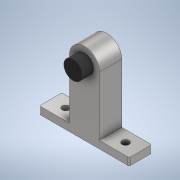
# Autodesk Inventor part: Stop sliding
Saved by Autodesk Inventor 2021 (Build 250183000, 183)
## iProperties
Created: 2021-06-07
Part Number: Stop sliding
Material: Generic
Document SubType Name: Modeling
Designer: Nelson
Density: 1 g/cm^3
Appearance: Default
Author: Nelson
Autodesk Inventor part; units mm, degrees
ref_plane "YZ Plane" through (0, 0, 0) normal (1, 0, 0) x (0, 1, 0)
ref_plane "XZ Plane" through (0, 0, 0) normal (0, 1, 0) x (-1, 0, 0)
ref_plane "XY Plane" through (0, 0, 0) normal (0, 0, 1) x (1, 0, 0)
sketch "Sketch3" plane through (0, 0, 0) normal (0, 0, 1) x (1, 0, 0)
  line L0 (0, 0) -> (60, 0)
  line L1 (60, 0) -> (60, 10)
  line L2 (60, 10) -> (20, 10)
  line L3 (20, 10) -> (20, 89)
  line L4 (0, 0) -> (0, 29.8306) construction
  line L5 (0, 0) -> (-60, 0)
  line L6 (-60, 0) -> (-60, 10)
  line L7 (-60, 10) -> (-20, 10)
  line L8 (-20, 10) -> (-20, 89)
  arc A0 (20, 89) -> (-20, 89) centre (0, 89) ccw
  dimension "d10" = 60
  dimension "d11" = 10
  dimension "d12" = 40
  dimension "d13" = 79
  dimension "d19" = 20
  constraints: 18 end point, 4 symmetric about line, 2 horizontal, 2 point on circle, 2 vertical, 1 centre point, 1 perpendicular
  measures "d10" distance of L0.start L0.end
  measures "d11" distance of L0.end L1.end
  measures "d12" distance of L1.end L2.end
  measures "d13" distance of L2.end L3.end
  measures "d19" radius of A0
extrude "Extrusion1" add sketch "Sketch3" against normal blind 30
sketch "Sketch4" plane through (0, 0, 0) normal (0, 0, 1) x (1, 0, 0)
  arc A0 (20, 89) -> (-20, 89) centre (0, 89) ccw projected
  circle A1 centre (0, 89) radius 12.5
  point P0 (0, 0)
  dimension "d20" = 25
  constraints: 1 centre point, 1 coincident
  measures "d20" diameter of A1
extrude "Extrusion2" add sketch "Sketch4" along normal blind 15
fillet "Fillet1" radius 2 4 edges at (60, 5, 0) (60, 5, -30) (-60, 5, 0) (-60, 5, -30)
sketch "Sketch5" plane through (-20, 10, 0) normal (0, 1, 0) x (1, 0, 0)
  line L0 (-38, 30) -> (0, 30) projected
  line L1 (40, 30) -> (78, 30) projected
  line L2 (-40, 2) -> (-40, 28) projected
  line L3 (80, 2) -> (80, 28) projected
  point P0 (20, 0)
  point P1 (-20, 15)
  point P2 (60, 15)
  dimension "d24" = 15
  dimension "d25" = 15
  dimension "d26" = 20
  dimension "d27" = 20
  measures "d24" distance from line of point (-20, 15) L0
  measures "d25" distance from line of L1 point (60, 15)
  measures "d26" distance from line of point (-20, 15) L2
  measures "d27" distance from line of point (60, 15) L3
hole "Hole1" at (-40, 10, -15) at (40, 10, -15) direction (0, -1, 0) diameter 9.5 depth 17.1 tip angle 137
equation "\"d27\" = d26"
body "Solid1"
